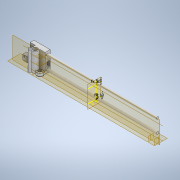
# Autodesk Inventor part: MKP2 - X Axis
Saved by Autodesk Inventor 2020.3 (Build 243373010, 373A)
## iProperties
Created: 2021-08-01
Part Number: MKP2 - X Axis
Material: Generic
Document SubType Name: Modeling
Designer: pepd9
Density: 1 g/cm^3
Appearance: Default
Author: pepd9
Autodesk Inventor part; units mm, degrees
ref_plane "Right Vertical Rod Plane" through (245, 0, 0) normal (1, 0, 0) x (0, 1, 0)
ref_plane "Left Vertical Rod Plane" through (-245, 0, 0) normal (1, 0, 0) x (0, 1, 0)
sketch "Sketch1" plane through (0, 0, 0) normal (0, 1, 0) x (-1, 0, 0)
  circle A0 centre (245, 0) radius 9.5
  circle A1 centre (245, 0) radius 13.5
  point P0 (0, 0)
  point P1 (-245, 0)
  dimension "d2" = 19
  dimension "d3" = 4
  constraints: 2 centre point, 1 coincident
  measures "d2" diameter of A0
  measures "d3" radial gap between concentric circles of A0 A1
extrude "Extrusion1" add sketch "Sketch1" along normal blind 80
ref_plane "Left Edge of Frame" through (-269, 0, 0) normal (1, 0, 0) x (0, 1, 0)
ref_plane "Right Edge of Frame" through (269, 0, 0) normal (1, 0, 0) x (0, 1, 0)
sketch "Sketch2" plane through (-245, 0, 0) normal (0, -1, 0) x (1, 0, 0)
  circle A0 centre (20, 0) radius 4
  circle A1 centre (20, 0) radius 12.5
  circle A2 centre (0, 0) radius 9.5 projected
  circle A3 centre (0, 0) radius 5 construction
  point P0 (245, 0)
  dimension "d10" = 8
  dimension "d11" = 25
  dimension "d12" = 10
  dimension "d13" = 20
  constraints: 3 centre point, 2 coincident
  measures "d10" diameter of A0
  measures "d11" diameter of A1
  measures "d12" diameter of A3
  measures "d13" distance of A2.centre A0.centre
extrude "Extrusion2" add sketch "Sketch2" along normal blind 4 separate body contours A1 A2 | A2 A1 picked at (11.7124, 4.0089) picked at (8.2303, 0)
sketch "Sketch3" plane through (-225, 0, 0) normal (0, 1, 0) x (1, 0, 0)
  circle A0 centre (0, 0) radius 4 projected
  circle A1 centre (0, 0) radius 6.5
  point P0 (225, 0)
  dimension "d16" = 13
  constraints: 1 centre point, 1 coincident
  measures "d16" diameter of A1
extrude "Extrusion3" add sketch "Sketch3" along normal blind 6 bodies 2
ref_plane "Horizontal Rod Plane Bottom" through (-245, 40, 0) normal (0, 1, 0) x (1, 0, 0)
ref_plane "Horizontal Rod Plane Top" through (-245, 67.5, 0) normal (0, 1, 0) x (1, 0, 0)
ref_plane "Work Plane10" through (-245, 12.5, 0) normal (0, 1, 0) x (1, 0, 0)
sketch "Sketch4" plane through (-225, -4, 0) normal (0, -1, 0) x (1, 0, 0)
  circle A0 centre (0, 0) radius 4 projected
  line L0 (-6.7175, -6.7175) -> (6.7175, -6.7175)
  line L1 (6.7175, -6.7175) -> (6.7175, 6.7175)
  line L2 (6.7175, 6.7175) -> (-6.7175, 6.7175)
  line L3 (-6.7175, 6.7175) -> (-6.7175, -6.7175)
  line L4 (-6.7175, -6.7175) -> (6.7175, 6.7175) construction
  line L5 (6.7175, -6.7175) -> (-6.7175, 6.7175) construction
  point P0 (225, 0)
  dimension "d44" = 19
  constraints: 12 end point, 2 midpoint, 2 parallel, 2 perpendicular, 1 horizontal
  measures "d44" distance of L0.start L1.end
hole "Hole1" at (-231.7175, -4, 6.7175) at (-218.2825, -4, 6.7175) at (-218.2825, -4, -6.7175) at (-231.7175, -4, -6.7175) direction (0, 1, 0) diameter 3.1 end through all bodies 2
chamfer "Chamfer1" distance 0.25 angle 45 11 edges at (-229, -4, 0) (-231.7175, -4, 8.2675) (-237.5, -4, 0) (-231.7175, 0, -5.1675) (-218.2825, 0, -5.1675) (-237.5, 0, 0) (-231.5, 6, 0) (-231.7175, 0, 8.2675) (-229, 6, 0) (-218.2825, 0, 8.2675) (-218.2825, -4, 8.2675)
sketch "Sketch5" plane through (0, 0, 0) normal (1, 0, 0) x (0, 1, 0)
  line L0 (80, -9.5) -> (0, -9.5) projected
  circle A0 centre (67.5, -18.5) radius 5
  line L1 (0, -13.5) -> (80, -13.5) projected
  line L2 (67.5, 21.5766) -> (67.5, -34.9594) projected
  circle A1 centre (12.5, -18.5) radius 5
  line L3 (12.5, 21.5766) -> (12.5, -34.9594) projected
  point P0 (0, 0)
  dimension "d33" = 10
  dimension "d34" = 0
  dimension "d35" = 10
  dimension "d36" = 0
  dimension "d37" = 5
  dimension "d38" = 5
  constraints: 2 centre point
  measures "d33" diameter of A0
  measures "d34" distance from line of L2 A0.centre
  measures "d35" diameter of A1
  measures "d36" distance from line of A1.centre L3
  measures "d37" distance from line of L1 A1.centre
  measures "d38" distance from line of L1 A0.centre
sketch "Sketch6" plane through (-225, 0, 0) normal (0, 1, 0) x (1, 0, 0)
  circle A0 centre (-20, 0) radius 13.5 projected
  circle A1 centre (0, 0) radius 4 projected
  circle A2 centre (0, 0) radius 14
  circle A3 centre (0, 0) radius 6.5 projected
  point P0 (225, 0)
  point P1 (-10.3438, -9.4343)
  point P2 (-10.3438, 9.4343)
  point P3 (-6.5, 0)
  dimension "d39" = 28
  constraints: 1 centre point, 1 coincident
  measures "d39" diameter of A2
extrude "Extrusion4" add sketch "Sketch6" along normal blind 10 contours A0 A2 picked at (11.366, 1.1103) bodies 1
sketch "Sketch7" plane through (0, 0, 0) normal (0, -1, 0) x (1, 0, 0)
  arc A0 (-235.3438, -9.4343) -> (-235.3438, 9.4343) centre (-225, 0) ccw projected
  line L0 (-211, -13.5) -> (-311, -13.5)
  line L1 (-311, -13.5) -> (-311, -29.5)
  line L2 (-311, -29.5) -> (-211, -29.5)
  line L3 (-211, -29.5) -> (-211, -13.5)
  line L4 (-211, 0) -> (-211, -13.5)
  arc A1 (-235.3438, -9.4343) -> (-235.3438, 9.4343) centre (-225, 0) ccw projected
  line L5 (-269, 22.4) -> (-269, -36.4) projected
  arc A2 (-235.3438, 9.4343) -> (-235.3438, -9.4343) centre (-245, 0) ccw projected
  line L6 (-258.5, 0) -> (-258.5, -13.5)
  circle A3 centre (-245, 0) radius 13.5 projected
  point P0 (0, 0)
  point P1 (-228.7081, -13.5)
  point P2 (-245, -13.5)
  point P3 (-221.2919, -13.5)
  dimension "d42" = 13.5
  dimension "d43" = 16
  dimension "d45" = 42
  constraints: 12 end point, 2 parallel, 2 perpendicular, 2 point on circle, 2 tangent, 1 horizontal, 1 point on line, 1 vertical, 1 vertical alignment
  measures "d42" distance from line of L0 A0.centre
  measures "d43" distance of L2.end L0.start
  measures "d45" distance between parallel lines of L5 L1
extrude "Extrusion5" add sketch "Sketch7" against normal up to surface (80 mm away) contours L0 L3 L2 L5 A0 | A2 L0 L6 | L0 A2 A0 | L2 L1 L0 L5 bodies 1
sketch "Sketch8" plane through (-311, 0, -13.5) normal (0, 0, 1) x (1, 0, 0)
  line L0 (5.5, 16) -> (36.5, 16)
  line L1 (36.5, 16) -> (36.5, 47)
  line L2 (36.5, 47) -> (5.5, 47)
  line L3 (5.5, 47) -> (5.5, 16)
  line L4 (52.5, 0) -> (52.5, 80) projected
  line L5 (0, 0) -> (0, 80) projected
  line L6 (-62.2, 0) -> (373.2, 0) projected
  line L7 (311, 7.5) -> (311, 17.5) projected
  line L8 (311, 12.5) -> (-154.6834, 12.5) construction
  point P0 (311, 0)
  dimension "d48" = 31
  dimension "d49" = 31
  dimension "d50" = 5.5
  dimension "d72" = 3.5
  constraints: 10 end point, 2 horizontal, 2 parallel, 1 perpendicular
  measures "d48" distance of L2.end L1.end
  measures "d49" distance of L1.end L0.end
  measures "d50" distance between parallel lines of L3 L5
  measures "d72" distance between parallel lines of L0 L8
hole "Hole2" at (-274.5, 47, -13.5) at (-305.5, 47, -13.5) at (-305.5, 16, -13.5) at (-274.5, 16, -13.5) direction (0, 0, -1) diameter 3.4 end through all counterbore diameter 6.5 counterbore depth 3 bodies 1 clearance for "Socket Head Cap Screw" size "M3" standard "Ansi Metric M Profile"
sketch "Sketch10" plane through (-311, 0, -29.5) normal (-1, 0, 0) x (0, 0, 1)
  line L0 (16, 50.25) -> (16, 43.75) projected
  line L1 (13, 43.75) -> (13, 50.25) projected
  line L2 (16, 19.25) -> (16, 12.75) projected
  line L3 (13, 12.75) -> (13, 19.25) projected
  line L4 (13, 45.3) -> (13, 48.7) projected
  line L5 (13, 47) -> (13, 16) construction
  line L6 (13, 14.3) -> (13, 17.7) projected
  line L7 (13, 31.5) -> (-16.6743, 31.5) construction
  line L8 (13.5, 41.5) -> (2.5, 41.5)
  line L9 (2.5, 41.5) -> (2.5, 21.5)
  line L10 (2.5, 21.5) -> (13.5, 21.5)
  line L11 (13.5, 21.5) -> (13.5, 41.5)
  line L12 (13.5, 41.5) -> (2.5, 21.5) construction
  line L13 (2.5, 41.5) -> (13.5, 21.5) construction
  line L14 (16, 0) -> (16, 80) projected
  line L15 (16, 31.5) -> (0, 31.5)
  line L16 (0, 0) -> (0, 80) projected
  point P0 (29.5, 0)
  point P1 (8, 31.5)
  point P2 (0, 56)
  point P3 (8, 31.5)
  dimension "d62" = 11
  dimension "d63" = 20
  constraints: 18 end point, 7 midpoint, 4 point on line, 2 horizontal, 2 parallel, 1 perpendicular
  measures "d62" distance of L10.end L9.end
  measures "d63" distance of L9.end L8.end
extrude "Extrusion7" cut sketch "Sketch10" against normal through all bodies 1
sketch "Sketch11" plane through (-311, 0, -13.5) normal (0, 0, 1) x (1, 0, 0)
  line L0 (0, 0) -> (0, 80) projected
  line L1 (52.5, 0) -> (0, 0) projected
  line L2 (52.5, 0) -> (52.5, 80) projected
  circle A0 centre (5.5, 16) radius 3.25 projected
  circle A1 centre (36.5, 47) radius 3.25 projected
  circle A2 centre (5.5, 47) radius 3.25 projected
  circle A3 centre (36.5, 16) radius 3.25 projected
  line L3 (5.5, 47) -> (36.5, 16)
  line L4 (11, 21.5) -> (31, 21.5)
  line L5 (31, 21.5) -> (31, 41.5)
  line L6 (31, 41.5) -> (11, 41.5)
  line L7 (11, 41.5) -> (11, 21.5)
  line L8 (11, 21.5) -> (31, 41.5) construction
  line L9 (31, 21.5) -> (11, 41.5) construction
  line L10 (52.5, 80) -> (0, 80) projected
  line L11 (0, 21.5) -> (100, 21.5) projected
  line L12 (11, 21.5) -> (0, 21.5)
  line L13 (31, 41.5) -> (31, 80)
  line L14 (52.5, 80) -> (0, 80) projected
  point P0 (311, 0)
  point P1 (21, 31.5)
  point P2 (0, 43.5)
  point P3 (31, 0)
  point P4 (31, 80)
  dimension "d66" = 20
  dimension "d67" = 20
  constraints: 18 end point, 3 midpoint, 3 point on line, 2 parallel, 2 perpendicular, 1 horizontal
  measures "d66" distance of L6.end L5.end
  measures "d67" distance of L5.end L4.end
extrude "Extrusion8" cut sketch "Sketch11" against normal through all contours L0 L10 L13 L6 L7 L11 | L7 L3 L4 | L3 L6 L5 | A2 bodies 1
sketch "Sketch12" plane through (-225, 10, 0) normal (0, 1, 0) x (1, 0, 0)
  arc A0 (-10.3438, -9.4343) -> (3.7081, 13.5) centre (0, 0) ccw projected
  line L0 (14, 13.5) -> (3.7081, 13.5) projected
  line L1 (14, 0) -> (14, 13.5)
  point P0 (225, 0)
  constraints: 2 end point, 1 point on circle, 1 vertical
extrude "Extrusion9" add sketch "Sketch12" against normal up to surface (10 mm away) bodies 1
sketch "Sketch13" plane through (0, 80, 0) normal (0, 1, 0) x (1, 0, 0)
  circle A0 centre (-245, 0) radius 9.5 projected
  line L0 (-280, 29.5) -> (-280, 13.5) projected
  line L1 (-258.5, 13.5) -> (-280, 13.5) projected
  line L2 (-258.5, 0) -> (-258.5, 13.5) projected
  arc A1 (-258.5, 0) -> (-235.3438, 9.4343) centre (-245, 0) ccw projected
  arc A2 (-221.2919, 13.5) -> (-235.3438, 9.4343) centre (-225, 0) ccw projected
  line L3 (-211, 13.5) -> (-221.2919, 13.5) projected
  line L4 (-211, 29.5) -> (-211, 13.5) projected
  line L5 (-280, 29.5) -> (-211, 29.5) projected
  line L6 (-245, 0) -> (-267.9132, -22.9132)
  circle A3 centre (-245, 0) radius 9.5 projected
  line L7 (-245, 0) -> (-271.896, 0)
  line L8 (-244.2929, -0.7071) -> (-267.2061, -23.6203)
  line L9 (-245.7071, 0.7071) -> (-268.6203, -22.2061)
  point P0 (0, 0)
  point P1 (-253.8126, -10.2268)
  point P2 (-250.9731, -7.3873)
  point P3 (-252.3873, -5.9731)
  point P4 (-255.2268, -8.8126)
  dimension "d73" = 45
  dimension "d74" = 1
  dimension "d75" = 1
  constraints: 8 end point, 2 parallel, 1 horizontal
  measures "d73" angle of L7 L6
  measures "d74" distance between parallel lines of L6 L8
  measures "d75" distance between parallel lines of L6 L9
extrude "Extrusion10" cut sketch "Sketch13" against normal through all contours L8 A1 L6 A0 | A0 L6 A1 L9 bodies 1
sketch "Sketch14" plane through (0, 80, 0) normal (0, 1, 0) x (1, 0, 0)
  line L0 (-250.9731, -7.3873) -> (-253.8126, -10.2268) projected
  arc A0 (-253.8126, -10.2268) -> (-235.3438, 9.4343) centre (-245, 0) ccw projected
  arc A1 (-221.2919, 13.5) -> (-235.3438, 9.4343) centre (-225, 0) ccw projected
  line L1 (-211, 13.5) -> (-221.2919, 13.5) projected
  line L2 (-211, 29.5) -> (-211, 13.5) projected
  line L3 (-280, 29.5) -> (-211, 29.5) projected
  line L4 (-280, 29.5) -> (-280, 13.5) projected
  line L5 (-258.5, 13.5) -> (-280, 13.5) projected
  line L6 (-258.5, 0) -> (-258.5, 13.5) projected
  arc A2 (-258.5, 0) -> (-255.2268, -8.8126) centre (-245, 0) ccw projected
  line L7 (-255.2268, -8.8126) -> (-252.3873, -5.9731) projected
  arc A3 (-250.9731, -7.3873) -> (-252.3873, -5.9731) centre (-245, 0) ccw projected
  line L8 (-250.9731, -7.3873) -> (-253.8126, -10.2268) projected
  line L9 (-250.9731, -7.3873) -> (-259.4695, -15.8837)
  line L10 (-259.4695, -15.8837) -> (-255.2268, -20.1263)
  line L11 (-255.2268, -20.1263) -> (-246.7304, -11.6299)
  line L12 (-246.7304, -11.6299) -> (-250.9731, -7.3873)
  line L13 (-252.3873, -5.9731) -> (-260.8837, -14.4695)
  line L14 (-260.8837, -14.4695) -> (-265.1263, -10.2268)
  line L15 (-265.1263, -10.2268) -> (-256.6299, -1.7304)
  line L16 (-256.6299, -1.7304) -> (-252.3873, -5.9731)
  point P0 (0, 0)
  point P1 (-248.2127, -13.1122)
  point P2 (-255.2268, -8.8126)
  point P3 (-258.1122, -3.2127)
  dimension "d78" = 6
  dimension "d79" = 6
  dimension "d80" = 8
  constraints: 16 end point, 4 parallel, 3 perpendicular, 2 point on line
  measures "d78" distance of L9.end L10.end
  measures "d79" distance of L13.end L14.end
  measures "d80" distance from line of L7.start L14
extrude "Extrusion11" add sketch "Sketch14" against normal up to surface (80 mm away) contours A0 L11 L10 L9 | L13 L14 L15 A2 bodies 1
sketch "Sketch15" plane through (0, 80, 0) normal (0, 1, 0) x (1, 0, 0)
  arc A0 (-231.5, 0) -> (-235.3438, 9.4343) centre (-245, 0) ccw projected
  circle A1 centre (-225, 0) radius 6.5 projected
  arc A2 (-235.3438, -9.4343) -> (-231.5, 0) centre (-245, 0) ccw projected
  arc A3 (-235.3438, -9.4343) -> (-211, 0) centre (-225, 0) ccw projected
  line L0 (-211, 0) -> (-211, 13.5) projected
  line L1 (-221.2919, 13.5) -> (-211, 13.5) projected
  arc A4 (-221.2919, 13.5) -> (-235.3438, 9.4343) centre (-225, 0) ccw projected
  line L2 (-211, 29.5) -> (-211, 0) projected
  line L3 (-211, 8.5) -> (-234.5119, 8.5)
  point P0 (0, 0)
  dimension "d85" = 2
  constraints: 2 end point, 1 horizontal alignment, 1 perpendicular, 1 point on circle, 1 point on line
extrude "Extrusion13" add sketch "Sketch15" against normal up to surface (70 mm away) contours A0 A4 L1 L0 L3 bodies 1
extrude "Extrusion12" cut sketch "Sketch5" against normal blind 255 contours A0 L2 | L2 A0 | A1 L3 | L3 A1 bodies 1
extrude "Extrusion14" add sketch "Sketch5" against normal mid plane 510 separate body contours A0 L2 | L2 A0
extrude "Extrusion15" add sketch "Sketch5" along normal mid plane 510 separate body contours A1 L3 | L3 A1
equation "\"d2\" = Bearing_OD"
equation "\"d33\" = Rod_Diameter"
equation "\"d35\" = Rod_Diameter"
equation "\"d0\" = 0.5 * Vertical_rod_distance"
equation "\"d1\" = -0.5 * Vertical_rod_distance"
equation "\"Rod_Diameter\" = 10"
equation "\"Clearance\" = 0.2"
equation "\"Bearing_OD\" = 19"
equation "\"Bearing_Length\" = 29"
equation "\"Horizontal_rod_spacing\" = 55"
equation "\"d19\" = 0.5 * Horizontal_rod_spacing"
equation "\"d20\" = -0.5 * Horizontal_rod_spacing"
equation "\"Vertical_rod_distance\" = 490"
body "Solid4"
